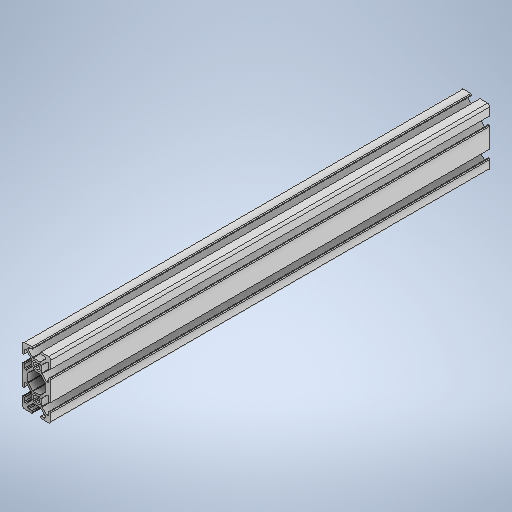
# Autodesk Inventor part: 20-40
Saved by Autodesk Inventor 2025 (Build 290162000, 162)
## iProperties
Created: 2024-06-18
Part Number: 20-40
Material: Generic
Document SubType Name: Modeling
Designer: mumin
Density: 1 g/cm^3
Appearance: Default
Author: mumin
Autodesk Inventor part; units mm, degrees
ref_plane "YZ Plane" through (0, 0, 0) normal (1, 0, 0) x (0, 1, 0)
ref_plane "XZ Plane" through (0, 0, 0) normal (0, 1, 0) x (-1, 0, 0)
ref_plane "XY Plane" through (0, 0, 0) normal (0, 0, 1) x (1, 0, 0)
sketch "Sketch1" plane through (0, 0, 0) normal (0, 0, 1) x (1, 0, 0)
  arc A0 (-8.5, -15.4946) -> (-7.992, -16.0026) centre (-7.992, -15.4946) ccw
  line L0 (-7.2659, -16.0026) -> (-7.992, -16.0026)
  arc A1 (-7.2659, -16.0026) -> (-6.9067, -15.8538) centre (-7.2659, -15.4946) ccw
  line L1 (-5.995, -17.9996) -> (-5.995, -17.2738)
  arc A2 (-5.8462, -16.9146) -> (-5.995, -17.2738) centre (-5.487, -17.2738) ccw
  arc A3 (-5.995, -17.9996) -> (-5.487, -18.5076) centre (-5.487, -17.9996) ccw
  line L2 (-3.8038, -12.7509) -> (-6.9067, -15.8538)
  line L3 (-8.5, -20.0076) -> (-3.138, -20.0076)
  line L4 (-3.138, -18.5076) -> (-5.487, -18.5076)
  arc A4 (-2.63, -19.0156) -> (-3.138, -18.5076) centre (-3.138, -19.0156) ccw
  line L5 (-2.63, -19.4996) -> (-2.63, -19.0156)
  arc A5 (-3.138, -20.0076) -> (-2.63, -19.4996) centre (-3.138, -19.4996) ccw
  line L6 (-5.8462, -16.9146) -> (-2.743, -13.8114)
  arc A6 (-8.5, -13.1456) -> (-9.008, -12.6376) centre (-9.008, -13.1456) ccw
  arc A7 (-9.492, -12.6376) -> (-10, -13.1456) centre (-9.492, -13.1456) ccw
  line L7 (-9.008, -12.6376) -> (-9.492, -12.6376)
  arc A8 (-10, -18.5076) -> (-8.5, -20.0076) centre (-8.5, -18.5076) ccw
  line L8 (-8.5, -15.4946) -> (-8.5, -13.1456)
  line L9 (-10, -13.1456) -> (-10, -18.5076)
  arc A9 (2.7433, -13.8114) -> (2.3841, -13.6626) centre (2.3841, -14.1706) ccw
  line L10 (2.7433, -13.8114) -> (5.8462, -16.9143)
  arc A10 (5.995, -17.2735) -> (5.8462, -16.9143) centre (5.487, -17.2735) ccw
  line L11 (5.995, -17.2735) -> (5.995, -17.9996)
  line L12 (7.992, -16.0026) -> (7.2662, -16.0026)
  arc A11 (6.907, -15.8538) -> (7.2662, -16.0026) centre (7.2662, -15.4946) ccw
  line L13 (6.907, -15.8538) -> (3.8038, -12.7506)
  arc A12 (7.992, -16.0026) -> (8.5, -15.4946) centre (7.992, -15.4946) ccw
  line L14 (10, -18.5076) -> (10, -13.1456)
  arc A13 (9.008, -12.6376) -> (8.5, -13.1456) centre (9.008, -13.1456) ccw
  line L15 (9.492, -12.6376) -> (9.008, -12.6376)
  arc A14 (10, -13.1456) -> (9.492, -12.6376) centre (9.492, -13.1456) ccw
  line L16 (8.5, -13.1456) -> (8.5, -15.4946)
  arc A15 (8.5, -20.0076) -> (10, -18.5076) centre (8.5, -18.5076) ccw
  arc A16 (5.487, -18.5076) -> (5.995, -17.9996) centre (5.487, -17.9996) ccw
  line L17 (5.487, -18.5076) -> (3.138, -18.5076)
  line L18 (3.138, -20.0076) -> (8.5, -20.0076)
  arc A17 (-2.3838, -13.6626) -> (-2.743, -13.8114) centre (-2.3838, -14.1706) ccw
  line L19 (-2.3838, -13.6626) -> (2.3841, -13.6626)
  line L20 (2.1245, -12.3121) -> (2.3045, -12.1321)
  arc A18 (2.3045, -12.1321) -> (1.9358, -10.8113) centre (1.748, -11.5756) ccw
  arc A19 (0.8037, -11.9434) -> (2.1245, -12.3121) centre (1.568, -11.7556) ccw
  arc A20 (-0.8037, -11.9434) -> (0.8037, -11.9434) centre (0, -10.0076) ccw
  line L21 (-2.3045, -12.1321) -> (-2.1245, -12.3121)
  arc A21 (-1.9358, -10.8113) -> (-2.3045, -12.1321) centre (-1.748, -11.5756) ccw
  arc A22 (-2.1245, -12.3121) -> (-0.8037, -11.9434) centre (-1.568, -11.7556) ccw
  arc A23 (3.8038, -7.2643) -> (3.655, -7.6235) centre (4.163, -7.6235) ccw
  arc A24 (2.3838, -6.3526) -> (2.743, -6.2038) centre (2.3838, -5.8446) ccw
  line L22 (3.8038, -7.2643) -> (6.9067, -4.1614)
  arc A25 (7.2659, -4.0126) -> (6.9067, -4.1614) centre (7.2659, -4.5206) ccw
  line L23 (5.995, -2.0156) -> (5.995, -2.7414)
  arc A26 (5.8462, -3.1006) -> (5.995, -2.7414) centre (5.487, -2.7414) ccw
  line L24 (7.2659, -4.0126) -> (7.992, -4.0126)
  arc A27 (8.5, -4.5206) -> (7.992, -4.0126) centre (7.992, -4.5206) ccw
  line L25 (10, -6.8696) -> (10, -1.5076)
  line L26 (8.5, -4.5206) -> (8.5, -6.8696)
  line L27 (5.8462, -3.1006) -> (2.743, -6.2038)
  arc A28 (3.655, -12.3914) -> (3.8038, -12.7506) centre (4.163, -12.3914) ccw
  line L28 (3.655, -12.3914) -> (3.655, -7.6235)
  line L29 (2.3045, -7.8831) -> (2.1245, -7.7031)
  arc A29 (2.1245, -7.7031) -> (0.8037, -8.0718) centre (1.568, -8.2596) ccw
  arc A30 (1.9358, -9.2039) -> (2.3045, -7.8831) centre (1.748, -8.4396) ccw
  arc A31 (0.8037, -8.0718) -> (-0.8037, -8.0718) centre (0, -10.0076) ccw
  arc A32 (1.9358, -10.8113) -> (1.9358, -9.2039) centre (0, -10.0076) ccw
  line L30 (2.3838, -6.3526) -> (-2.3841, -6.3526)
  line L31 (-2.7433, -6.2038) -> (-5.8462, -3.1009)
  arc A33 (-5.995, -2.7417) -> (-5.8462, -3.1009) centre (-5.487, -2.7417) ccw
  line L32 (-5.995, -2.7417) -> (-5.995, -0.0076)
  arc A34 (-6.907, -4.1614) -> (-7.2662, -4.0126) centre (-7.2662, -4.5206) ccw
  arc A35 (-7.992, -4.0126) -> (-8.5, -4.5206) centre (-7.992, -4.5206) ccw
  line L33 (-6.907, -4.1614) -> (-3.8038, -7.2646)
  line L34 (-10, -1.5076) -> (-10, -6.8696)
  line L35 (-8.5, -6.8696) -> (-8.5, -4.5206)
  arc A36 (-9.008, -7.3776) -> (-8.5, -6.8696) centre (-9.008, -6.8696) ccw
  line L36 (-9.492, -7.3776) -> (-9.008, -7.3776)
  arc A37 (-10, -6.8696) -> (-9.492, -7.3776) centre (-9.492, -6.8696) ccw
  line L37 (-7.992, -4.0126) -> (-7.2662, -4.0126)
  line L38 (-5.571, -0.0076) -> (-5.995, -0.0076)
  arc A38 (-2.7433, -6.2038) -> (-2.3841, -6.3526) centre (-2.3841, -5.8446) ccw
  arc A39 (-3.655, -7.6238) -> (-3.8038, -7.2646) centre (-4.163, -7.6238) ccw
  arc A40 (-3.8038, -12.7509) -> (-3.655, -12.3917) centre (-4.163, -12.3917) ccw
  arc A41 (8.5, -6.8696) -> (9.008, -7.3776) centre (9.008, -6.8696) ccw
  line L39 (9.008, -7.3776) -> (9.492, -7.3776)
  arc A42 (9.492, -7.3776) -> (10, -6.8696) centre (9.492, -6.8696) ccw
  arc A43 (3.138, -18.5076) -> (2.63, -19.0156) centre (3.138, -19.0156) ccw
  line L40 (2.63, -19.0156) -> (2.63, -19.4996)
  arc A44 (2.63, -19.4996) -> (3.138, -20.0076) centre (3.138, -19.4996) ccw
  line L41 (-2.1245, -7.7031) -> (-2.3045, -7.8831)
  arc A45 (-2.3045, -7.8831) -> (-1.9358, -9.2039) centre (-1.748, -8.4396) ccw
  arc A46 (-0.8037, -8.0718) -> (-2.1245, -7.7031) centre (-1.568, -8.2596) ccw
  line L42 (-3.655, -7.6238) -> (-3.655, -12.3917)
  arc A47 (-1.9358, -9.2039) -> (-1.9358, -10.8113) centre (0, -10.0076) ccw
  arc A48 (-8.5, 19.9924) -> (-10, 18.4924) centre (-8.5, 18.4924) ccw
  line L43 (-8.5, 19.9924) -> (-3.138, 19.9924)
  line L44 (-3.138, 18.4924) -> (-5.487, 18.4924)
  arc A49 (-3.138, 18.4924) -> (-2.63, 19.0004) centre (-3.138, 19.0004) ccw
  line L45 (-2.63, 19.4844) -> (-2.63, 19.0004)
  arc A50 (-2.63, 19.4844) -> (-3.138, 19.9924) centre (-3.138, 19.4844) ccw
  arc A51 (-9.008, 12.6224) -> (-8.5, 13.1304) centre (-9.008, 13.1304) ccw
  line L46 (-9.008, 12.6224) -> (-9.492, 12.6224)
  arc A52 (-10, 13.1304) -> (-9.492, 12.6224) centre (-9.492, 13.1304) ccw
  line L47 (-2.3045, 12.1169) -> (-2.1245, 12.2969)
  arc A53 (-2.3045, 12.1169) -> (-1.9358, 10.7961) centre (-1.748, 11.5604) ccw
  arc A54 (-1.9358, 10.7961) -> (-1.9358, 9.1887) centre (0, 9.9924) ccw
  arc A55 (-1.9358, 9.1887) -> (-2.3045, 7.8679) centre (-1.748, 8.4244) ccw
  line L48 (-2.1245, 7.6879) -> (-2.3045, 7.8679)
  line L49 (-3.655, 7.6086) -> (-3.655, 12.3765)
  arc A56 (-3.8038, 7.2494) -> (-3.655, 7.6086) centre (-4.163, 7.6086) ccw
  arc A57 (5.8462, 16.8991) -> (5.995, 17.2583) centre (5.487, 17.2583) ccw
  line L50 (5.995, 17.2583) -> (5.995, 17.9844)
  arc A58 (5.995, 17.9844) -> (5.487, 18.4924) centre (5.487, 17.9844) ccw
  line L51 (3.138, 19.9924) -> (8.5, 19.9924)
  line L52 (5.487, 18.4924) -> (3.138, 18.4924)
  arc A59 (2.63, 19.0004) -> (3.138, 18.4924) centre (3.138, 19.0004) ccw
  line L53 (2.63, 19.0004) -> (2.63, 19.4844)
  arc A60 (3.138, 19.9924) -> (2.63, 19.4844) centre (3.138, 19.4844) ccw
  line L54 (7.992, 15.9874) -> (7.2662, 15.9874)
  arc A61 (7.2662, 15.9874) -> (6.907, 15.8386) centre (7.2662, 15.4794) ccw
  arc A62 (10, 18.4924) -> (8.5, 19.9924) centre (8.5, 18.4924) ccw
  arc A63 (8.5, 15.4794) -> (7.992, 15.9874) centre (7.992, 15.4794) ccw
  line L55 (10, 18.4924) -> (10, 13.1304)
  line L56 (8.5, 13.1304) -> (8.5, 15.4794)
  arc A64 (8.5, 13.1304) -> (9.008, 12.6224) centre (9.008, 13.1304) ccw
  line L57 (9.492, 12.6224) -> (9.008, 12.6224)
  arc A65 (9.492, 12.6224) -> (10, 13.1304) centre (9.492, 13.1304) ccw
  arc A66 (-2.743, 13.7962) -> (-2.3838, 13.6474) centre (-2.3838, 14.1554) ccw
  line L58 (-2.3838, 13.6474) -> (2.3841, 13.6474)
  arc A67 (0.8037, 11.9282) -> (-0.8037, 11.9282) centre (0, 9.9924) ccw
  arc A68 (-0.8037, 11.9282) -> (-2.1245, 12.2969) centre (-1.568, 11.7404) ccw
  arc A69 (2.1245, 12.2969) -> (0.8037, 11.9282) centre (1.568, 11.7404) ccw
  line L59 (2.1245, 12.2969) -> (2.3045, 12.1169)
  arc A70 (1.9358, 10.7961) -> (2.3045, 12.1169) centre (1.748, 11.5604) ccw
  arc A71 (1.9358, 9.1887) -> (1.9358, 10.7961) centre (0, 9.9924) ccw
  arc A72 (3.8038, 12.7354) -> (3.655, 12.3762) centre (4.163, 12.3762) ccw
  arc A73 (2.3045, 7.8679) -> (1.9358, 9.1887) centre (1.748, 8.4244) ccw
  line L60 (2.3045, 7.8679) -> (2.1245, 7.6879)
  line L61 (3.655, 12.3762) -> (3.655, 7.6083)
  arc A74 (3.655, 7.6083) -> (3.8038, 7.2491) centre (4.163, 7.6083) ccw
  line L62 (5.995, -2.0156) -> (5.995, 2.7262)
  arc A75 (5.995, 2.7262) -> (5.8462, 3.0854) centre (5.487, 2.7262) ccw
  line L63 (7.2659, 3.9974) -> (7.992, 3.9974)
  arc A76 (6.9067, 4.1462) -> (7.2659, 3.9974) centre (7.2659, 4.5054) ccw
  line L64 (5.8462, 3.0854) -> (2.743, 6.1886)
  line L65 (3.8038, 7.2491) -> (6.9067, 4.1462)
  arc A77 (7.992, 3.9974) -> (8.5, 4.5054) centre (7.992, 4.5054) ccw
  line L66 (10, 6.8544) -> (10, -6.8696)
  line L67 (8.5, 4.5054) -> (8.5, 6.8544)
  arc A78 (0.8037, 8.0566) -> (2.1245, 7.6879) centre (1.568, 8.2444) ccw
  arc A79 (2.743, 6.1886) -> (2.3838, 6.3374) centre (2.3838, 5.8294) ccw
  arc A80 (-0.8037, 8.0566) -> (0.8037, 8.0566) centre (0, 9.9924) ccw
  line L68 (2.3838, 6.3374) -> (-2.3841, 6.3374)
  arc A81 (-2.1245, 7.6879) -> (-0.8037, 8.0566) centre (-1.568, 8.2444) ccw
  arc A82 (-2.3841, 6.3374) -> (-2.7433, 6.1886) centre (-2.3841, 5.8294) ccw
  arc A83 (9.008, 7.3624) -> (8.5, 6.8544) centre (9.008, 6.8544) ccw
  line L69 (9.008, 7.3624) -> (9.492, 7.3624)
  arc A84 (10, 6.8544) -> (9.492, 7.3624) centre (9.492, 6.8544) ccw
  line L70 (-2.7433, 6.1886) -> (-5.8462, 3.0857)
  arc A85 (-5.8462, 3.0857) -> (-5.995, 2.7265) centre (-5.487, 2.7265) ccw
  arc A86 (-8.5, 4.5054) -> (-7.992, 3.9974) centre (-7.992, 4.5054) ccw
  line L71 (-10, -6.8696) -> (-10, 6.8544)
  line L72 (-6.907, 4.1462) -> (-3.8038, 7.2494)
  line L73 (-7.992, 3.9974) -> (-7.2662, 3.9974)
  arc A87 (-7.2662, 3.9974) -> (-6.907, 4.1462) centre (-7.2662, 4.5054) ccw
  line L74 (-5.995, 2.7265) -> (-5.995, -0.0076)
  line L75 (-8.5, 6.8544) -> (-8.5, 4.5054)
  arc A88 (-8.5, 6.8544) -> (-9.008, 7.3624) centre (-9.008, 6.8544) ccw
  line L76 (-9.492, 7.3624) -> (-9.008, 7.3624)
  arc A89 (-9.492, 7.3624) -> (-10, 6.8544) centre (-9.492, 6.8544) ccw
  arc A90 (-7.992, 15.9874) -> (-8.5, 15.4794) centre (-7.992, 15.4794) ccw
  arc A91 (-5.487, 18.4924) -> (-5.995, 17.9844) centre (-5.487, 17.9844) ccw
  line L77 (-5.995, 17.9844) -> (-5.995, 17.2586)
  arc A92 (-5.995, 17.2586) -> (-5.8462, 16.8994) centre (-5.487, 17.2586) ccw
  arc A93 (-6.9067, 15.8386) -> (-7.2659, 15.9874) centre (-7.2659, 15.4794) ccw
  line L78 (-5.8462, 16.8994) -> (-2.743, 13.7962)
  arc A94 (-3.655, 12.3765) -> (-3.8038, 12.7357) centre (-4.163, 12.3765) ccw
  line L79 (-3.8038, 12.7357) -> (-6.9067, 15.8386)
  line L80 (-7.2659, 15.9874) -> (-7.992, 15.9874)
  line L81 (-10, 13.1304) -> (-10, 18.4924)
  line L82 (-8.5, 15.4794) -> (-8.5, 13.1304)
  arc A95 (2.3841, 13.6474) -> (2.7433, 13.7962) centre (2.3841, 14.1554) ccw
  line L83 (2.7433, 13.7962) -> (5.8462, 16.8991)
  line L84 (6.907, 15.8386) -> (3.8038, 12.7354)
  point P0 (0, 0)
  point P1 (0, -10.0076)
  point P2 (-5.995, -2.0156)
  point P3 (0, -0.0152)
  point P4 (0, 9.9924)
  constraints: 192 point on circle, 170 end point, 96 centre point, 3 point on line
extrude "Extrusion1" add sketch "Sketch1" along normal mid plane 304.8
body "Solid1"
